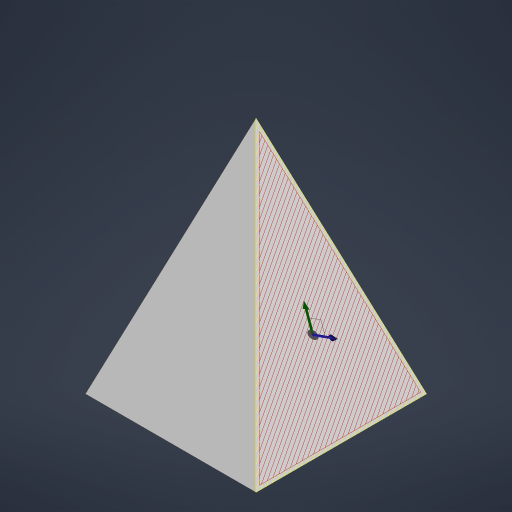
# Autodesk Inventor part: exp1
Saved by Autodesk Inventor 2023 (Build 270158000, 158)
## iProperties
Created: 2023-03-11
Part Number: exp1
Material: Generic
Document SubType Name: Modeling
Designer: kamraj
Density: 1 g/cm^3
Appearance: Default
Author: kamraj
Autodesk Inventor part; units mm, degrees
ref_plane "YZ Plane" through (0, 0, 0) normal (1, 0, 0) x (0, 1, 0)
ref_plane "XZ Plane" through (0, 0, 0) normal (0, 1, 0) x (-1, 0, 0)
ref_plane "XY Plane" through (0, 0, 0) normal (0, 0, 1) x (1, 0, 0)
sketch "Sketch3" plane through (0, 0, 0) normal (0, 1, 0) x (-1, 0, 0)
  line L0 (-25, 25) -> (25, 25)
  line L1 (25, 25) -> (25, -25)
  line L2 (25, -25) -> (-25, -25)
  line L3 (-25, -25) -> (-25, 25)
  line L4 (-25, 25) -> (25, -25) construction
  line L5 (25, 25) -> (-25, -25) construction
  point P0 (0, 0)
  dimension "d6" = 50
  dimension "d7" = 50
  constraints: 12 end point, 2 midpoint, 2 parallel, 1 horizontal, 1 perpendicular
  measures "d6" distance of L1.end L2.end
  measures "d7" distance of L0.end L1.end
extrude "Extrusion2" add sketch "Sketch3" along normal blind 70
sketch "Sketch4" plane through (-25, 0, 25) normal (0, 0, 1) x (1, 0, 0)
  line L0 (50, 0) -> (0, 0) projected
  line L1 (0, 0) -> (25, 70)
  line L2 (50, 70) -> (0, 70) projected
  line L3 (0, 0) -> (0, 70) projected
  line L4 (0, 70) -> (0, 0)
  point P0 (25, 0)
  constraints: 4 end point, 1 collinear, 1 midpoint
extrude "Extrusion3" cut sketch "Sketch4" along normal through all both and the other way through all
mirror "Mirror1" about plane through (0, 0, 0) normal (1, 0, 0) of "Extrusion3"
sketch "Sketch5" plane through (0, 0, 0) normal (1, 0, 0) x (0, 1, 0)
  line L0 (70, -25) -> (70, 25) projected
  line L1 (70, 0) -> (70, -25)
  line L2 (70, -25) -> (0, -25)
  line L3 (0, -25) -> (70, 0)
  point P0 (0, 0)
  constraints: 6 end point, 1 midpoint, 1 perpendicular, 1 vertical
extrude "Extrusion4" cut sketch "Sketch5" along normal through all both and the other way through all
mirror "Mirror2" about plane through (0, 0, 0) normal (0, 0, 1) of "Extrusion4"
body "Solid2"
